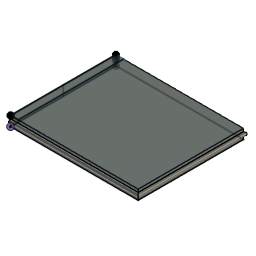
lid (Autodesk Fusion 360 design; units mm, degrees)
part number: 2026-02-18-21-48-13-710
Autodesk Fusion 360 part; units mm, degrees
sketch "Sketch1" plane through (0, 0, 0) normal (0, 0, 1) x (1, 0, 0)
  line L0 (0, 0) -> (26.4, 0)
  line L1 (26.4, 0) -> (26.4, 21.8)
  line L2 (26.4, 21.8) -> (0, 21.8)
  line L3 (0, 21.8) -> (0, 0)
  dimension "d1" = 26.4
  dimension "d2" = 21.8
  constraint horizontal L0
  constraint vertical L1
  constraint horizontal L2
  constraint vertical L3
  constraint coincident L0.start L3.end
  measures "d1" distance of L0.start L0.end
  measures "d2" distance of L0.start L2.end
extrude "Extrude1" add sketch "Sketch1" along normal blind 2
sketch "Sketch2" plane through (0, 0, 0) normal (-1, 0, 0) x (0, -1, 0)
  line L0 (-21.8, 0) -> (0, 0)
  line L1 (0, 0) -> (0, 2)
  line L2 (0, 2) -> (-21.8, 2)
  line L3 (-21.8, 2) -> (-21.8, 0)
  line L4 (-21.8, 2) -> (-21.8, 0) construction
  line L5 (0, 0) -> (-21.8, 0)
  line L6 (0, 0) -> (0, 2) construction
  line L7 (0, 2) -> (-21.8, 2)
  arc A0 (-21.8, 1.4) -> (-21.8, 0.6) centre (-21.8, 1) ccw
  line L8 (-10.9, 2) -> (-10.9, 0)
  line L9 (-21.8, 2) -> (-21.8, 1.4)
  line L10 (-21.8, 0.6) -> (-21.8, 0)
  dimension "d5" = 0.4
  constraint coincident L2.end L3.start
  constraint coincident L0.start L3.end
  constraint coincident L0.end L1.start
  constraint coincident L1.end L2.start
  constraint coincident L3 A0.start
  constraint midpoint L3 A0.centre
  constraint coincident L4 A0.end
  constraint midpoint L7 L8.start
  constraint midpoint L5 L8.end
  measures "d5" radius of A0
sweep "Sweep1" add profiles "Sketch2" along 3 edges at (13.2, 0, 2) (26.4, 10.9, 2) (13.2, 21.8, 2) section 1 contours L3 A0
sketch "Sketch3" plane through (0, 0, 0) normal (-1, 0, 0) x (0, -1, 0)
sketch "Sketch4" plane through (0, 0, 2) normal (0, 0, 1) x (-1, 0, 0)
  line L0 (0, -21.8) -> (0, 0)
  line L1 (0, 0) -> (-26.4, 0)
  line L2 (-26.4, 0) -> (-26.4, -21.8)
  line L3 (-26.4, -21.8) -> (0, -21.8)
  line L4 (0, 0) -> (-1.6, 0)
  line L5 (-1.6, 0) -> (-1.6, -21.7864)
  line L6 (-1.6, -21.7864) -> (0, -21.7864)
  line L7 (0, -21.7864) -> (0, 0)
  dimension "d12" = 1.6
  constraint horizontal L4
  constraint vertical L5
  constraint horizontal L6
  constraint vertical L7
  constraint coincident L0.end L1.start
  measures "d12" distance of L0.end L4.end
